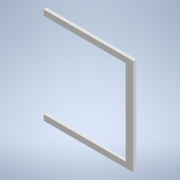
# Autodesk Inventor part: pcb_holder_5
Saved by Autodesk Inventor 2020 (Build 240168000, 168)
## iProperties
Created: 2019-08-29
Part Number: pcb_holder_5
Material: Generic
Document SubType Name: Modeling
Designer: psrob
Density: 1 g/cm^3
Appearance: Default
Author: psrob
Autodesk Inventor part; units mm, degrees
ref_plane "YZ Plane" through (0, 0, 0) normal (1, 0, 0) x (0, 1, 0)
ref_plane "XZ Plane" through (0, 0, 0) normal (0, 1, 0) x (-1, 0, 0)
ref_plane "XY Plane" through (0, 0, 0) normal (0, 0, 1) x (1, 0, 0)
sketch "Sketch1" plane through (0, 0, 0) normal (0, 0, 1) x (1, 0, 0)
  circle A0 centre (24.4575, -9.7625) radius 0.65 projected
  circle A1 centre (24.4575, -14.7625) radius 0.65 projected
  circle A2 centre (-17.4525, 9.4575) radius 0.65 projected
  circle A3 centre (-17.4525, 14.4575) radius 0.65 projected
  circle A4 centre (-17.4525, -3.2525) radius 0.65 projected
  circle A5 centre (-17.4525, 1.7475) radius 0.65 projected
  circle A6 centre (-17.4525, -16.5825) radius 0.65 projected
  circle A7 centre (-17.4525, -11.5825) radius 0.65 projected
  circle A8 centre (23.1875, -0.1525) radius 0.51 projected
  circle A9 centre (23.1875, 2.3875) radius 0.51 projected
  circle A10 centre (23.1875, 4.9275) radius 0.51 projected
  circle A11 centre (23.1875, 7.4675) radius 0.51 projected
  circle A12 centre (23.1875, 11.2775) radius 0.51 projected
  circle A13 centre (23.1875, 13.8175) radius 0.51 projected
  circle A14 centre (23.1875, 16.3575) radius 0.51 projected
  circle A15 centre (23.1875, 18.8975) radius 0.51 projected
  circle A16 centre (2.8675, 17.6275) radius 0.51 projected
  circle A17 centre (5.4075, 17.6275) radius 0.51 projected
  circle A18 centre (7.9475, 17.6275) radius 0.51 projected
  circle A19 centre (10.4875, 17.6275) radius 0.51 projected
  circle A20 centre (13.0275, 17.6275) radius 0.51 projected
  circle A21 centre (15.5675, 17.6275) radius 0.51 projected
  circle A22 centre (-6.6575, -12.8525) radius 0.5 projected
  circle A23 centre (-6.6575, 0.4825) radius 0.5 projected
  circle A24 centre (-6.6575, 13.1825) radius 0.5 projected
  circle A25 centre (10.4875, 13.8175) radius 0.5 projected
  circle A26 centre (16.8375, 3.6575) radius 0.5 projected
  circle A27 centre (5.4075, 13.8175) radius 0.5 projected
  circle A28 centre (1.5975, 11.2775) radius 0.5 projected
  circle A29 centre (7.9475, 13.8175) radius 0.5 projected
  circle A30 centre (1.5975, 8.7375) radius 0.5 projected
  circle A31 centre (1.5975, 6.1975) radius 0.5 projected
  circle A32 centre (16.8375, 6.1975) radius 0.5 projected
  circle A33 centre (16.8375, 11.2775) radius 0.5 projected
  circle A34 centre (9.2175, -16.6625) radius 0.5 projected
  circle A35 centre (13.0275, 13.8175) radius 0.5 projected
  circle A36 centre (16.8375, 8.7375) radius 0.5 projected
  circle A37 centre (1.5975, 3.6575) radius 0.5 projected
  circle A38 centre (2.8675, 13.8175) radius 0.5 projected
  circle A39 centre (16.8375, -9.0425) radius 0.5 projected
  circle A40 centre (16.8375, -11.5825) radius 0.5 projected
  circle A41 centre (16.8375, -14.1225) radius 0.5 projected
  circle A42 centre (16.8375, -16.6625) radius 0.5 projected
  circle A43 centre (1.5975, -16.6625) radius 0.5 projected
  circle A44 centre (1.5975, -14.1225) radius 0.5 projected
  circle A45 centre (1.5975, -11.5825) radius 0.5 projected
  circle A46 centre (1.5975, -9.0425) radius 0.5 projected
  circle A47 centre (1.5975, -6.5025) radius 0.5 projected
  circle A48 centre (1.5975, -3.9625) radius 0.5 projected
  circle A49 centre (1.5975, -1.4225) radius 0.5 projected
  circle A50 centre (1.5975, 1.1175) radius 0.5 projected
  circle A51 centre (15.5675, 13.8175) radius 0.5 projected
  circle A52 centre (14.2975, -16.6625) radius 0.5 projected
  circle A53 centre (11.7575, -16.6625) radius 0.5 projected
  circle A54 centre (14.2975, 2.3875) radius 0.5 projected
  circle A55 centre (14.2975, -0.1525) radius 0.5 projected
  circle A56 centre (16.8375, 1.1175) radius 0.5 projected
  circle A57 centre (16.8375, -1.4225) radius 0.5 projected
  circle A58 centre (16.8375, -3.9625) radius 0.5 projected
  circle A59 centre (16.8375, -6.5025) radius 0.5 projected
  circle A60 centre (6.6775, -7.7725) radius 0.175 projected
  circle A61 centre (-22.6821, 5.5625) radius 0.175 projected
  circle A62 centre (-24.2879, 8.7375) radius 0.175 projected
  circle A63 centre (5.09, -6.6613) radius 0.175 projected
  circle A64 centre (-2.0537, -14.1225) radius 0.175 projected
  circle A65 centre (-17.4525, -5.8675) radius 0.175 projected
  circle A66 centre (-18.5729, -6.9493) radius 0.175 projected
  circle A67 centre (-14.2775, -7.3937) radius 0.175 projected
  circle A68 centre (-14.2775, -9.0425) radius 0.175 projected
  circle A69 centre (-2.3712, 13.8175) radius 0.175 projected
  circle A70 centre (-2.53, -8.725) radius 0.175 projected
  circle A71 centre (-0.9425, -6.6613) radius 0.175 projected
  circle A72 centre (2.3913, -10.1537) radius 0.175 projected
  circle A73 centre (-0.3075, -10.1537) radius 0.175 projected
  circle A74 centre (-16.6587, 5.5625) radius 0.175 projected
  circle A75 centre (-10.9437, 6.515) radius 0.175 projected
  circle A76 centre (-20.8815, 13.0555) radius 0.175 projected
  circle A77 centre (-21.8975, -12.8525) radius 0.175 projected
  circle A78 centre (-21.8975, -1.4225) radius 0.175 projected
  circle A79 centre (-21.8975, 10.0075) radius 0.175 projected
  circle A80 centre (-4.7525, 3.34) radius 0.175 projected
  circle A81 centre (-4.7525, -9.995) radius 0.175 projected
  circle A82 centre (-19.3575, 17.6275) radius 0.175 projected
  circle A83 centre (-25.0725, -11.5825) radius 0.175 projected
  circle A84 centre (-25.0725, -0.1525) radius 0.175 projected
  circle A85 centre (-25.0725, 11.2775) radius 0.175 projected
  line L0 (-28.2475, -22.3775) -> (28.2475, -22.3775) projected
  line L1 (28.2475, -22.3775) -> (28.2475, 22.3775) projected
  line L2 (28.2475, 22.3775) -> (-28.2475, 22.3775) projected
  line L3 (-28.2475, 22.3775) -> (-28.2475, -22.3775) projected
  line L4 (28.2475, 22.3775) -> (28.7475, 22.3775)
  line L5 (28.7475, 22.3775) -> (28.7475, 22.8775)
  line L6 (28.7475, 22.8775) -> (28.2475, 22.8775)
  line L7 (28.2475, 22.8775) -> (28.2475, 22.3775)
  line L8 (28.2475, -22.3775) -> (28.7475, -22.3775)
  line L9 (28.7475, -22.3775) -> (28.7475, -22.8775)
  line L10 (28.7475, -22.8775) -> (28.2475, -22.8775)
  line L11 (28.2475, -22.8775) -> (28.2475, -22.3775)
  line L12 (28.7475, 22.8775) -> (32.7475, 22.8775)
  line L13 (32.7475, 22.8775) -> (32.7475, -22.8775)
  line L14 (32.7475, -22.8775) -> (28.7475, -22.8775)
  line L15 (28.7475, -22.8775) -> (28.7475, 22.8775)
  line L16 (32.7475, 22.8775) -> (-15.2525, 22.8775)
  line L17 (-15.2525, 22.8775) -> (-15.2525, 25.8775)
  line L18 (-15.2525, 25.8775) -> (32.7475, 25.8775)
  line L19 (32.7475, 25.8775) -> (32.7475, 22.8775)
  line L20 (32.7475, -22.8775) -> (-15.2525, -22.8775)
  line L21 (-15.2525, -22.8775) -> (-15.2525, -25.8775)
  line L22 (-15.2525, -25.8775) -> (32.7475, -25.8775)
  line L23 (32.7475, -25.8775) -> (32.7475, -22.8775)
  point P0 (0, 0)
  dimension "d0" = 0.5
  dimension "d1" = 0.5
  dimension "d2" = 0.5
  dimension "d3" = 0.5
  dimension "d4" = 4
  dimension "d5" = 45.755
  dimension "d6" = 48
  dimension "d7" = 3
  dimension "d8" = 48
  dimension "d9" = 3
  constraints: 40 end point, 10 parallel, 5 horizontal, 5 perpendicular
  measures "d0" distance of L6.end L5.end
  measures "d1" distance of L5.end L4.end
  measures "d2" distance of L9.end L10.end
  measures "d3" distance of L8.end L9.end
  measures "d4" distance of L13.end L14.end
  measures "d5" distance of L12.end L13.end
  measures "d6" distance of L17.end L18.end
  measures "d7" distance of L16.end L17.end
  measures "d8" distance of L22.end L21.end
  measures "d9" distance of L21.end L20.end
ref_plane "Work Plane1" through (-28.2475, -22.3775, -1.6) normal (0, 0, -1) x (0, 1, 0)
extrude "Extrusion1" add sketch "Sketch1" against normal up to surface (1.6 mm away) contours L15 L5 L12 L13 L14 L9 | L10 L14 L23 L22 L21 L20 | L16 L17 L18 L19 L12 L6
sketch "Sketch2" plane through (0, 0, 0) normal (0, 0, 1) x (1, 0, 0)
  line L0 (28.7475, 22.8775) -> (28.7475, -22.8775) projected
  line L1 (28.7475, -22.8775) -> (-15.2525, -22.8775) projected
  line L2 (-15.2525, -22.8775) -> (-15.2525, -25.8775) projected
  line L3 (-15.2525, -25.8775) -> (32.7475, -25.8775) projected
  line L4 (32.7475, -25.8775) -> (32.7475, 25.8775) projected
  line L5 (32.7475, 25.8775) -> (-15.2525, 25.8775) projected
  line L6 (-15.2525, 25.8775) -> (-15.2525, 22.8775) projected
  line L7 (-15.2525, 22.8775) -> (28.7475, 22.8775) projected
  line L8 (-28.2475, 22.3775) -> (-28.2475, -22.3775) projected
  line L9 (-15.2525, -22.8775) -> (-15.2525, -25.8775) projected
  line L10 (-15.2525, -25.8775) -> (-28.2475, -25.8775)
  line L11 (-28.2475, -25.8775) -> (-28.2475, -22.8775)
  line L12 (-28.2475, -22.8775) -> (-15.2525, -22.8775)
  line L13 (-15.2525, -22.8775) -> (-15.2525, -25.8775)
  point P0 (0, 0)
  constraints: 8 end point, 2 parallel, 1 horizontal, 1 perpendicular
extrude "Extrusion2" add sketch "Sketch2" against normal up to surface (1.6 mm away) contours L2 L10 L11 L12
sketch "Sketch3" plane through (0, 0, 0) normal (0, 0, 1) x (1, 0, 0)
  line L0 (28.7475, 22.8775) -> (28.7475, -22.8775) projected
  line L1 (28.7475, -22.8775) -> (-28.2475, -22.8775) projected
  line L2 (-28.2475, -22.8775) -> (-28.2475, -25.8775) projected
  line L3 (-28.2475, -25.8775) -> (32.7475, -25.8775) projected
  line L4 (32.7475, -25.8775) -> (32.7475, 25.8775) projected
  line L5 (32.7475, 25.8775) -> (-15.2525, 25.8775) projected
  line L6 (-15.2525, 25.8775) -> (-15.2525, 22.8775) projected
  line L7 (-15.2525, 22.8775) -> (28.7475, 22.8775) projected
  line L8 (-28.2475, 22.3775) -> (-28.2475, -22.3775) projected
  line L9 (-28.2475, -22.3775) -> (28.2475, -22.3775) projected
  line L10 (-28.2475, -22.8775) -> (-28.2475, -25.8775) projected
  line L11 (-28.2475, -22.8775) -> (-31.2475, -22.8775)
  line L12 (-31.2475, -22.8775) -> (-31.2475, -19.8775)
  line L13 (28.7475, -22.8775) -> (-28.2475, -22.8775) projected
  line L14 (-31.2475, -19.8775) -> (-28.2475, -22.8775)
  line L15 (-31.2475, -19.8775) -> (-33.2475, -19.8775)
  line L16 (-33.2475, -19.8775) -> (-33.2475, -25.8775)
  line L17 (-33.2475, -25.8775) -> (-28.2475, -25.8775)
  point P0 (0, 0)
  dimension "d14" = 3
  dimension "d15" = 3
  dimension "d16" = 2
  constraints: 12 end point, 3 perpendicular, 2 horizontal
  measures "d14" distance of L1.end L11.end
  measures "d15" distance of L11.end L12.end
  measures "d16" distance of L12.end L15.end
extrude "Extrusion3" add sketch "Sketch3" against normal up to surface (1.6 mm away) contours L2 L17 L16 L15 L12 L11 | L11 L12 L14
ref_plane "Work Plane2" through (32.7475, 0, -1.6) normal (0, -1, 0) x (1, 0, 0)
sketch "Sketch4" plane through (0, 0, 0) normal (0, 0, 1) x (1, 0, 0)
  line L0 (28.7475, 22.8775) -> (28.7475, -22.8775) projected
  line L1 (28.7475, -22.8775) -> (-28.2475, -22.8775) projected
  line L2 (-28.2475, -22.8775) -> (-31.2475, -19.8775) projected
  line L3 (-31.2475, -19.8775) -> (-33.2475, -19.8775) projected
  line L4 (-33.2475, -19.8775) -> (-33.2475, -25.8775) projected
  line L5 (-33.2475, -25.8775) -> (32.7475, -25.8775) projected
  line L6 (32.7475, -25.8775) -> (32.7475, 25.8775) projected
  line L7 (32.7475, 25.8775) -> (-15.2525, 25.8775) projected
  line L8 (-15.2525, 25.8775) -> (-15.2525, 22.8775) projected
  line L9 (-15.2525, 22.8775) -> (28.7475, 22.8775) projected
  line L10 (-33.2475, -25.8775) -> (28.7475, -25.8775)
  line L11 (28.7475, -25.8775) -> (28.7475, -21.3775)
  line L12 (28.7475, -21.3775) -> (-33.2475, -21.3775)
  line L13 (-33.2475, -21.3775) -> (-33.2475, -25.8775)
  point P0 (0, 0)
  dimension "d19" = 61.995
  dimension "d20" = 4.5
  constraints: 8 end point, 2 parallel, 1 horizontal, 1 perpendicular
  measures "d19" distance of L12.end L11.end
  measures "d20" distance of L11.end L10.end
extrude "Extrusion4" add sketch "Sketch4" along normal blind 1.5 contours L0 L1 L2 L12 | L11 L5 L4 L12 L2 L1
sketch "Sketch5" plane through (32.7475, 25.8775, -1.6) normal (0, 0, -1) x (-1, 0, 0)
  line L0 (65.995, -47.255) -> (65.995, -51.755) projected
  line L1 (65.995, -51.755) -> (4, -51.755) projected
  line L2 (4, -51.755) -> (4, -47.255) projected
  line L3 (4, -47.255) -> (65.995, -47.255) projected
  point P0 (32.7475, -25.8775)
extrude "Extrusion5" add sketch "Sketch5" along normal blind 1.5
sketch "Sketch6" plane through (0, 0, 0) normal (0, 0, 1) x (1, 0, 0)
  line L0 (28.7475, -22.8775) -> (28.7475, -25.8775) projected
  line L1 (28.7475, -25.8775) -> (32.7475, -25.8775) projected
  line L2 (32.7475, -25.8775) -> (32.7475, 25.8775) projected
  line L3 (32.7475, 25.8775) -> (-15.2525, 25.8775) projected
  line L4 (-15.2525, 25.8775) -> (-15.2525, 22.8775) projected
  line L5 (-15.2525, 22.8775) -> (28.7475, 22.8775) projected
  line L6 (28.7475, 22.8775) -> (28.7475, -21.3775) projected
  line L7 (28.7475, -21.3775) -> (28.7475, -22.8775) projected
  line L8 (32.7475, 25.8775) -> (-15.2525, 25.8775) projected
  line L9 (-15.2525, 25.8775) -> (-2.2525, 25.8775)
  line L10 (-2.2525, 25.8775) -> (12.7475, 25.8775)
  line L11 (12.7475, 25.8775) -> (12.7475, 18.8775)
  line L12 (12.7475, 18.8775) -> (-2.2525, 18.8775)
  line L13 (-2.2525, 18.8775) -> (-2.2525, 25.8775)
  point P0 (0, 0)
  dimension "d25" = 13
  dimension "d26" = 15
  dimension "d27" = 7
  constraints: 10 end point, 2 parallel, 1 horizontal, 1 perpendicular, 1 point on line
  measures "d25" distance of L3.end L9.end
  measures "d26" distance of L11.end L12.end
  measures "d27" distance of L10.end L11.end
extrude "Extrusion6" add sketch "Sketch6" along normal blind 1.5 contours L11 L12 L13 L5 | L5 L13 L3 L11
sketch "Sketch7" plane through (32.7475, 25.8775, -1.6) normal (0, 0, -1) x (-1, 0, 0)
  line L0 (35, -3) -> (20, -3) projected
  line L1 (20, -7) -> (20, -3) projected
  line L2 (35, -7) -> (20, -7) projected
  line L3 (35, -3) -> (35, -7) projected
  line L4 (20, 0) -> (20, -3) projected
  line L5 (35, -3) -> (35, 0) projected
  line L6 (35, 0) -> (20, 0)
  point P0 (32.7475, -25.8775)
  constraints: 2 end point, 1 horizontal
extrude "Extrusion7" add sketch "Sketch7" along normal blind 1.5
chamfer "Chamfer1" distance 4 angle 45 4 edges at (12.7475, 18.8775, 0.75) (-2.2525, 18.8775, 0.75) (-2.2525, 18.8775, -2.35) (12.7475, 18.8775, -2.35)
body "Solid1"
